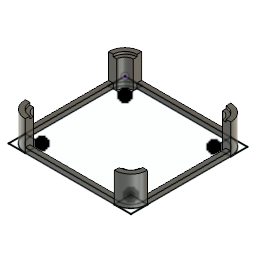
test_bench (Autodesk Fusion 360 design; units mm, degrees)
Autodesk Fusion 360 part; units mm, degrees
sketch "Sketch1" plane through (0, 0, 0) normal (0, 0, 1) x (1, 0, 0)
  line L0 (0, 0) -> (103, 0)
  line L1 (103, 0) -> (103, -98)
  line L2 (103, -98) -> (0, -98)
  line L3 (0, -98) -> (0, 0)
  line L4 (4, -84) -> (4, -14)
  line L5 (14, -4) -> (89, -4)
  line L6 (99, -14) -> (99, -84)
  line L7 (89, -94) -> (14, -94)
  arc A0 (14, -4) -> (4, -14) centre (14, -14) ccw
  arc A1 (99, -14) -> (89, -4) centre (89, -14) ccw
  arc A2 (4, -84) -> (14, -94) centre (14, -84) ccw
  arc A3 (89, -94) -> (99, -84) centre (89, -84) ccw
  line L8 (0, 0) -> (14, 0)
  line L9 (14, 0) -> (14, -14)
  line L10 (14, -14) -> (0, -14)
  line L11 (0, -14) -> (0, 0)
  line L12 (103, 0) -> (89, 0)
  line L13 (89, 0) -> (89, -14)
  line L14 (89, -14) -> (103, -14)
  line L15 (103, -14) -> (103, 0)
  line L16 (0, -98) -> (14, -98)
  line L17 (14, -98) -> (14, -84)
  line L18 (14, -84) -> (0, -84)
  line L19 (0, -84) -> (0, -98)
  line L20 (103, -98) -> (89, -98)
  line L21 (89, -98) -> (89, -84)
  line L22 (89, -84) -> (103, -84)
  line L23 (103, -84) -> (103, -98)
  arc A4 (14, 0) -> (0, -14) centre (14, -14) ccw
  arc A5 (103, -14) -> (89, 0) centre (89, -14) ccw
  arc A6 (89, -98) -> (103, -84) centre (89, -84) ccw
  arc A7 (0, -84) -> (14, -98) centre (14, -84) ccw
  dimension "d4" = 10
  dimension "d5" = 10
  dimension "d6" = 10
  dimension "d7" = 10
  dimension "d15" = 70
  dimension "d17" = 75
  constraint horizontal L0
  constraint vertical L1
  constraint horizontal L2
  constraint vertical L3
  constraint coincident L0.start L3.end
  constraint tangent L4 A0
  constraint tangent L5 A0
  constraint tangent L5 A1
  constraint tangent L6 A1
  constraint tangent L4 A2
  constraint tangent L7 A2
  constraint tangent L6 A3
  constraint tangent L7 A3
  constraint horizontal L8
  constraint vertical L9
  constraint horizontal L10
  constraint vertical L11
  constraint coincident A0.centre L9.end
  constraint horizontal L12
  constraint vertical L13
  constraint horizontal L14
  constraint vertical L15
  constraint coincident A1.centre L13.end
  constraint horizontal L16
  constraint vertical L17
  constraint horizontal L18
  constraint vertical L19
  constraint coincident A2.centre L17.end
  constraint horizontal L20
  constraint vertical L21
  constraint horizontal L22
  constraint vertical L23
  constraint coincident A3.centre L21.end
  constraint tangent L11 A4
  constraint tangent L1 A5
  constraint tangent L23 A6
  constraint tangent L16 A7
  measures "d4" radius of A0
  measures "d5" radius of A1
  measures "d6" radius of A2
  measures "d7" radius of A3
  measures "d15" distance of L10 L18
  measures "d17" distance of L9 L13
extrude "Extrude1" add sketch "Sketch1" along normal blind 4 contours L0 L5 L9 L13 | A0 L9 L10 A4 | L3 L4 L10 L18 | A1 L13 L14 A5 | A0 L9 L10 | A2 L17 L18 A7 | A1 L13 L14 | L1 L6 L14 L22 | A2 L17 L18 | L2 L7 L17 L21 | A3 L21 L22 A6 | A3 L21 L22
extrude "Extrude2" add sketch "Sketch1" along normal blind 25 contours A0 L9 L10 A4 | A1 L13 L14 A5 | A0 L9 L10 | A2 L17 L18 A7 | A1 L13 L14 | A2 L17 L18 | A3 L21 L22 A6 | A3 L21 L22
sketch "Sketch2" plane through (0, 0, 25) normal (0, 0, 1) x (-1, 0, 0)
  line L0 (-14, 14) -> (-14, 0)
  arc A0 (-14, 0) -> (0, 14) centre (-14, 14) ccw
  line L1 (0, 14) -> (-14, 14)
  arc A1 (-14, 4) -> (-4, 14) centre (-14, 14) ccw
  line L2 (-14, 0) -> (-14, 14)
  line L3 (-14, 14) -> (0, 14)
  arc A2 (-14, 0) -> (0, 14) centre (-14, 14) ccw
  arc A3 (-103, 14) -> (-89, 0) centre (-89, 14) ccw
  arc A4 (-99, 14) -> (-89, 4) centre (-89, 14) ccw
  line L4 (-89, 0) -> (-89, 14)
  line L5 (-89, 14) -> (-103, 14)
  line L6 (-14, 84) -> (0, 84)
  line L7 (-14, 98) -> (-14, 84)
  arc A5 (-4, 84) -> (-14, 94) centre (-14, 84) ccw
  arc A6 (0, 84) -> (-14, 98) centre (-14, 84) ccw
  line L8 (-89, 84) -> (-103, 84)
  line L9 (-89, 98) -> (-89, 84)
  arc A7 (-89, 94) -> (-99, 84) centre (-89, 84) ccw
  arc A8 (-89, 98) -> (-103, 84) centre (-89, 84) ccw
extrude "Extrude3" cut sketch "Sketch2" against normal blind 2 contours L0 L1 A1 L2 L3 | A4 L4 L5 | L6 L7 A5 | L8 L9 A7
sketch "Sketch3" plane through (0, 0, 23) normal (0, 0, 1) x (-1, 0, 0)
  arc A0 (-14, 4) -> (-4, 14) centre (-14, 14) ccw
  line L0 (-4, 14) -> (-14, 14)
  line L1 (-14, 14) -> (-14, 4)
  circle A1 centre (-14, 14) radius 7
  circle A2 centre (-89, 14) radius 7
  circle A3 centre (-14, 84) radius 7
  circle A4 centre (-89, 84) radius 7
  dimension "d14" = 14
  dimension "d20" = -75
  dimension "d21" = 70
  constraint concentric A0 A1
  measures "d14" diameter of A1
extrude "Extrude4" cut sketch "Sketch3" against normal up to surface (23 mm away) contours L0 L1 A1 | A2 | A3 | A4 picked at (-12.3733, 9.6387)
